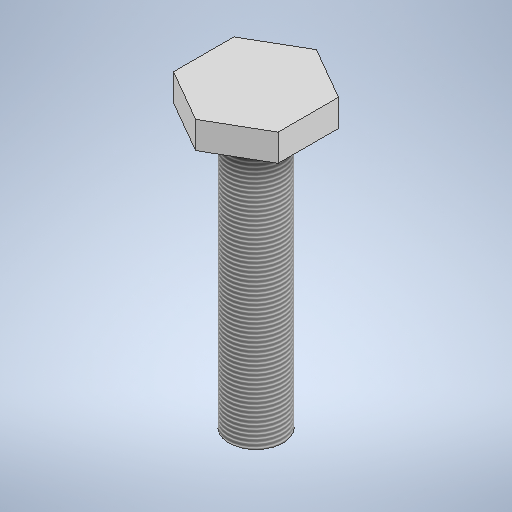
# Autodesk Inventor part: pe_parafuso
Saved by Autodesk Inventor 2025.2 (Build 292293000, 293)
## iProperties
Created: 2025-04-08
Part Number: pe_parafuso
Material: Generic
Document SubType Name: Modeling
Designer: kenne
Density: 1 g/cm^3
Appearance: Default
Author: kenne
Autodesk Inventor part; units mm, degrees
ref_plane "YZ Plane" through (0, 0, 0) normal (1, 0, 0) x (0, 1, 0)
ref_plane "XZ Plane" through (0, 0, 0) normal (0, 1, 0) x (-1, 0, 0)
ref_plane "XY Plane" through (0, 0, 0) normal (0, 0, 1) x (1, 0, 0)
sketch "Sketch1" plane through (0, 0, 0) normal (0, 0, 1) x (1, 0, 0)
  line L0 (0, 5) -> (0, -5)
  line L1 (-1, -5) -> (0, -5)
  line L2 (-1, -5) -> (-1, 5)
  line L3 (-1, 5) -> (0, 5)
  point P0 (0, 0)
  dimension "d0" = 10
  dimension "d1" = 1
  constraints: 8 end point, 2 horizontal, 2 vertical, 1 horizontal alignment, 1 midpoint
  measures "d0" distance of L0.start L0.end
  measures "d1" distance of L1.start L0.end
revolve "Revolution1" add sketch "Sketch1" angle 360 about axis through (0, 5, 0) along (0, -1, 0)
sketch "Sketch2" plane through (0, 5, 0) normal (0, 1, 0) x (1, 0, 0)
  line L0 (1.9365, -1.118) -> (0, -2.2361)
  line L1 (0, -2.2361) -> (-1.9365, -1.118)
  line L2 (-1.9365, -1.118) -> (-1.9365, 1.118)
  line L3 (-1.9365, 1.118) -> (0, 2.2361)
  line L4 (0, 2.2361) -> (1.9365, 1.118)
  line L5 (1.9365, 1.118) -> (1.9365, -1.118)
  point P0 (0, 0)
  point P1 (0, 0)
  dimension "d3" = 1.9365
  constraints: 12 end point, 1 coincident, 1 vertical alignment, 13 other
  measures "d3" distance from line of point (0, 0) L4
extrude "Extrusion1" add sketch "Sketch2" along normal blind 1
thread "Thread1" size "M0.6x0.15" class "6g" standard "ANSI Metric M Profile" full length
body "Solid1"
